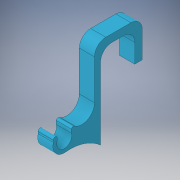
# Autodesk Inventor part: Curtain Adapter
Saved by Autodesk Inventor 2017 (Build 210142000, 142)
## iProperties
Created: 2016-10-24
Part Number: Curtain Adapter
Material: Generic
Document SubType Name: Modeling
Designer: andrew
Density: 1 g/cm^3
Appearance: Turquoise
Author: andrew
Autodesk Inventor part; units mm, degrees
ref_plane "YZ Plane" through (0, 0, 0) normal (1, 0, 0) x (0, 1, 0)
ref_plane "XZ Plane" through (0, 0, 0) normal (0, 1, 0) x (-1, 0, 0)
ref_plane "XY Plane" through (0, 0, 0) normal (0, 0, 1) x (1, 0, 0)
sketch "Sketch1" plane through (0, 0, 0) normal (1, 0, 0) x (0, 1, 0)
  line L0 (-57.15, 14.351) -> (12.7, 14.351)
  line L1 (12.7, 14.351) -> (12.7, -14.351)
  line L2 (12.7, -14.351) -> (-12.7, -14.351)
  line L3 (-12.7, -14.351) -> (-12.7, -20.701)
  line L4 (-12.7, -20.701) -> (19.05, -20.701)
  line L5 (19.05, -20.701) -> (19.05, 19.431)
  line L6 (19.05, 19.431) -> (-23.8064, 19.431)
  arc A0 (-36.322, 50.927) -> (-36.322, 38.735) centre (-38.1, 44.831) ccw
  arc A1 (-36.322, 50.927) -> (-31.3296, 51.5467) centre (-34.544, 57.023) ccw
  arc A2 (-35.433, 53.975) -> (-47.5727, 43.8339) centre (-38.1, 44.831) ccw
  arc A3 (-57.15, 14.351) -> (-47.5727, 43.8339) centre (-85.4633, 39.8454) ccw
  arc A4 (-35.433, 53.975) -> (-32.9368, 54.2848) centre (-34.544, 57.023) ccw
  line L7 (-32.9368, 54.2848) -> (-31.3296, 51.5467)
  arc A5 (-31.3296, 38.1153) -> (-36.322, 38.735) centre (-34.544, 32.639) ccw
  line L8 (-31.3296, 38.1153) -> (-32.9368, 35.3772)
  line L9 (-38.1, 44.831) -> (-26.6352, 44.831) construction
  arc A6 (-32.9368, 35.3772) -> (-23.8064, 19.431) centre (-23.8064, 30.018) ccw
  point P0 (0, 0)
  point P1 (12.7, 0)
  dimension "d0" = 5.08
  dimension "d1" = 3.175
  dimension "d2" = 38.1
  dimension "d3" = 6.35
  dimension "d5" = 6.35
  dimension "d7" = 50.8
  dimension "d8" = 6.35
  dimension "d9" = 6.35
  dimension "d11" = 19.05
  dimension "d12" = 12.7
  dimension "d13" = 25.4
  dimension "d14" = 28.702
  dimension "d15" = 6.35
  dimension "d16" = 12.192
  dimension "d17" = 25.4
  constraints: 20 end point, 14 point on circle, 7 centre point, 6 perpendicular, 6 tangent, 3 vertical alignment, 2 coincident, 2 horizontal, 1 equal length, 1 horizontal alignment, 1 midpoint, 1 point on line, 1 other
  measures "d0" distance between parallel lines of L0 L6
  measures "d1" radial gap between concentric circles of A2 A0
  measures "d2" radius of A3
  measures "d3" radius of A1
  measures "d5" radius of A0
  measures "d7" distance from line of L1 A0.centre
  measures "d8" distance between parallel lines of L5 L1
  measures "d9" distance between parallel lines of L2 L4
  measures "d11" horizontal distance of L0.start A0.centre
  measures "d12" distance from line of point (0, 0) L1
  measures "d13" distance of L1.end L2.end
  measures "d14" distance of L0.end L1.end
  measures "d15" radius of A5
  measures "d16" distance of A0.end A0.start
  measures "d17" distance between parallel lines of L6 L9
extrude "Extrusion1" add sketch "Sketch1" along normal blind 12.7
fillet "Fillet1" radius 9.525 4 edges at (6.35, 12.7, 14.351) (6.35, 12.7, -14.351) (6.35, 19.05, 19.431) (6.35, 19.05, -20.701)
fillet "Fillet2" radius 1.5875 3 edges at (6.35, -31.3296, 51.5467) (6.35, -32.9368, 54.2848) (6.35, -31.3296, 38.1153)
equation "\"d15\" = d3"
equation "\"d16\" = 1.92 * d5"
body "Solid1"
